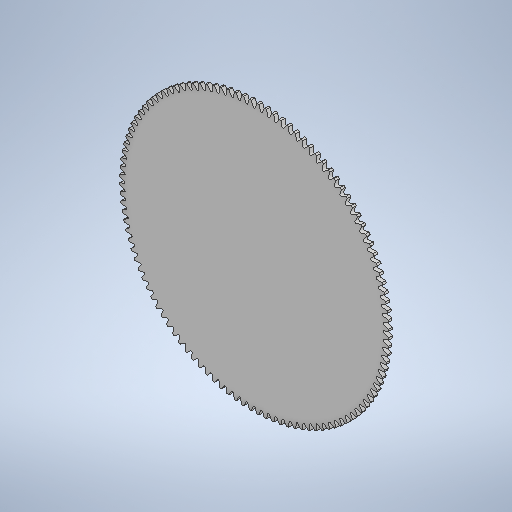
# Autodesk Inventor part: big gear 2.0
Saved by Autodesk Inventor 2025 (Build 290162010, 162A)
## iProperties
Created: 2025-09-06
Part Number: big gear 2.0
Material: Generic
Document SubType Name: Modeling
Designer: pokla
Density: 1 g/cm^3
Appearance: Default
Author: pokla
Autodesk Inventor part; units mm, degrees
ref_plane "YZ Plane" through (0, 0, 0) normal (1, 0, 0) x (0, 1, 0)
ref_plane "XZ Plane" through (0, 0, 0) normal (0, 1, 0) x (-1, 0, 0)
ref_plane "XY Plane" through (0, 0, 0) normal (0, 0, 1) x (1, 0, 0)
sketch "Sketch1" plane through (0, 0, 0) normal (0, 0, 1) x (1, 0, 0)
  spline S0 degree 3 poles (-14.9165, 712.3438) (-14.3601, 711.0686) (-13.2474, 708.5182) (-11.6564, 704.6592) (-10.1258, 700.7761) (-8.6597, 696.8679) (-7.2786, 692.9293) (-6.2598, 689.9687) (-5.6659, 687.9678) (-5.3327, 687.1621) (-4.9908, 686.5548) (-4.6754, 686.1384) (-4.3362, 685.7407) (-3.9402, 685.3992) (-3.5213, 685.0871) (-2.9134, 684.7464) (-2.2513, 684.5144) (-1.5656, 684.391) (-0.8692, 684.3646) (0, 684.3819) (0.8692, 684.3646) (1.5656, 684.391) (2.2513, 684.5144) (2.9134, 684.7464) (3.5213, 685.0871) (3.9402, 685.3992) (4.3362, 685.7407) (4.6754, 686.1384) (4.9908, 686.5548) (5.3327, 687.1621) (5.6659, 687.9678) (6.2598, 689.9687) (7.2786, 692.9293) (8.6597, 696.8679) (10.1258, 700.7761) (11.6564, 704.6592) (13.2474, 708.5182) (14.3601, 711.0686) (14.9165, 712.3438) knots 0 0 0 0 0.417378 0.834757 1.252136 1.669514 2.086891 2.50427 2.608615 2.712858 2.765031 2.8172 2.869347 2.921514 2.97367 3.025847 3.130039 3.182219 3.234379 3.338724 3.443069 3.495228 3.547409 3.6516 3.703778 3.755934 3.808101 3.860247 3.912416 3.964589 4.068833 4.173177 4.590556 5.007934 5.425312 5.842691 6.260069 6.677448 6.677448 6.677448 6.677448
  circle A0 centre (0, 0) radius 684.375 construction
  circle A1 centre (0, 0) radius 657.7848 construction
  circle A2 centre (0, 0) radius 700 construction
  circle A3 centre (0, 0) radius 712.5
  point P0 (-13.2604, 708.5127)
  point P1 (-11.6665, 704.6552)
  point P2 (-10.1366, 700.7719)
  point P3 (-8.6739, 696.8628)
  point P4 (-7.2824, 692.9279)
  point P5 (-5.9656, 688.9672)
  point P6 (-5.6486, 687.9731)
  point P7 (-5.2411, 687.0136)
  point P8 (-4.981, 686.5614)
  point P9 (-4.6714, 686.1415)
  point P10 (-4.3267, 685.7501)
  point P11 (-3.9363, 685.4041)
  point P12 (-3.5151, 685.0965)
  point P13 (-3.0605, 684.8405)
  point P14 (-2.0783, 684.4927)
  point P15 (-1.5643, 684.4032)
  point P16 (-1.0434, 684.3746)
  point P17 (0, 684.375)
  point P18 (1.0434, 684.3746)
  point P19 (1.5643, 684.4032)
  point P20 (2.0783, 684.4927)
  point P21 (3.0605, 684.8405)
  point P22 (3.5151, 685.0965)
  point P23 (3.9363, 685.4041)
  point P24 (4.3267, 685.7501)
  point P25 (4.6714, 686.1415)
  point P26 (4.981, 686.5614)
  point P27 (5.2411, 687.0136)
  point P28 (5.6486, 687.9731)
  point P29 (5.9656, 688.9672)
  point P30 (7.2824, 692.9279)
  point P31 (8.6739, 696.8628)
  point P32 (10.1366, 700.7719)
  point P33 (11.6665, 704.6552)
  point P34 (13.2604, 708.5127)
  constraints: 4 centre point, 2 point on circle, 79 other
extrude "Extrusion1" add sketch "Sketch1" against normal blind 20
extrude "Extrusion2" cut sketch "Sketch1" against normal through all contours A3 S0 picked at (-0.9229, 701.9967)
pattern_circular "Circular Pattern1" count 112 over 360 about axis through (0, 0, -10) along (0, 0, 1) of "Extrusion2"
sketch "Sketch2" plane through (0, 0, 0) normal (0, 0, 1) x (1, 0, 0)
  circle A0 centre (0, 0) radius 360
  line L0 (0, 0) -> (0, 360) construction
  line L1 (0, 0) -> (76.6258, 680.0718)
  line L2 (0, 0) -> (-76.6258, 680.0718)
  arc A1 (25.0484, 712.0596) -> (14.9165, 712.3438) centre (0, 0) ccw projected
  arc A2 (-14.9165, 712.3438) -> (-25.0484, 712.0596) centre (0, 0) ccw projected
  arc A3 (-54.8344, 710.3868) -> (-64.9345, 709.5349) centre (0, 0) ccw projected
  arc A4 (-94.5799, 706.1947) -> (-104.6163, 704.7778) centre (0, 0) ccw projected
  arc A5 (-134.0277, 699.7805) -> (-143.9689, 697.8031) centre (0, 0) ccw projected
  arc A6 (-173.0539, 691.1647) -> (-182.8686, 688.6329) centre (0, 0) ccw projected
  arc A7 (-211.5356, 680.3741) -> (-221.1928, 677.2961) centre (0, 0) ccw projected
  arc A8 (-249.3517, 667.4429) -> (-258.8212, 663.8282) centre (0, 0) ccw projected
  arc A9 (-286.3832, 652.4116) -> (-295.6351, 648.2716) centre (0, 0) ccw projected
  arc A10 (-322.5137, 635.3276) -> (-331.5189, 630.6754) centre (0, 0) ccw projected
  arc A11 (-357.6294, 616.2446) -> (-366.3596, 611.0948) centre (0, 0) ccw projected
  arc A12 (-391.6199, 595.2227) -> (-400.0476, 589.5915) centre (0, 0) ccw projected
  arc A13 (-424.3782, 572.328) -> (-432.4769, 566.2331) centre (0, 0) ccw projected
  arc A14 (-455.8013, 547.6326) -> (-463.5455, 541.0931) centre (0, 0) ccw projected
  arc A15 (-485.7902, 521.2141) -> (-493.1556, 514.2507) centre (0, 0) ccw projected
  arc A16 (-514.2507, 493.1556) -> (-521.2141, 485.7902) centre (0, 0) ccw projected
  arc A17 (-541.0931, 463.5455) -> (-547.6326, 455.8013) centre (0, 0) ccw projected
  arc A18 (-566.2331, 432.4769) -> (-572.328, 424.3782) centre (0, 0) ccw projected
  arc A19 (-589.5915, 400.0476) -> (-595.2227, 391.6199) centre (0, 0) ccw projected
  arc A20 (-611.0948, 366.3596) -> (-616.2446, 357.6294) centre (0, 0) ccw projected
  arc A21 (-630.6754, 331.5189) -> (-635.3276, 322.5137) centre (0, 0) ccw projected
  arc A22 (-648.2716, 295.6351) -> (-652.4116, 286.3832) centre (0, 0) ccw projected
  arc A23 (-663.8282, 258.8212) -> (-667.4429, 249.3517) centre (0, 0) ccw projected
  arc A24 (-677.2961, 221.1928) -> (-680.3741, 211.5356) centre (0, 0) ccw projected
  arc A25 (-688.6329, 182.8686) -> (-691.1647, 173.0539) centre (0, 0) ccw projected
  arc A26 (-697.8031, 143.9689) -> (-699.7805, 134.0277) centre (0, 0) ccw projected
  arc A27 (-704.7778, 104.6163) -> (-706.1947, 94.5799) centre (0, 0) ccw projected
  arc A28 (-709.5349, 64.9345) -> (-710.3868, 54.8344) centre (0, 0) ccw projected
  arc A29 (-712.0596, 25.0484) -> (-712.3438, 14.9165) centre (0, 0) ccw projected
  arc A30 (-712.3438, -14.9165) -> (-712.0596, -25.0484) centre (0, 0) ccw projected
  arc A31 (-710.3868, -54.8344) -> (-709.5349, -64.9345) centre (0, 0) ccw projected
  arc A32 (-706.1947, -94.5799) -> (-704.7778, -104.6163) centre (0, 0) ccw projected
  arc A33 (-699.7805, -134.0277) -> (-697.8031, -143.9689) centre (0, 0) ccw projected
  arc A34 (-691.1647, -173.0539) -> (-688.6329, -182.8686) centre (0, 0) ccw projected
  arc A35 (-680.3741, -211.5356) -> (-677.2961, -221.1928) centre (0, 0) ccw projected
  arc A36 (-667.4429, -249.3517) -> (-663.8282, -258.8212) centre (0, 0) ccw projected
  arc A37 (-652.4116, -286.3832) -> (-648.2716, -295.6351) centre (0, 0) ccw projected
  arc A38 (-635.3276, -322.5137) -> (-630.6754, -331.5189) centre (0, 0) ccw projected
  arc A39 (-616.2446, -357.6294) -> (-611.0948, -366.3596) centre (0, 0) ccw projected
  arc A40 (-595.2227, -391.6199) -> (-589.5915, -400.0476) centre (0, 0) ccw projected
  arc A41 (-572.328, -424.3782) -> (-566.2331, -432.4769) centre (0, 0) ccw projected
  arc A42 (-547.6326, -455.8013) -> (-541.0931, -463.5455) centre (0, 0) ccw projected
  arc A43 (-521.2141, -485.7902) -> (-514.2507, -493.1556) centre (0, 0) ccw projected
  arc A44 (-493.1556, -514.2507) -> (-485.7902, -521.2141) centre (0, 0) ccw projected
  arc A45 (-463.5455, -541.0931) -> (-455.8013, -547.6326) centre (0, 0) ccw projected
  arc A46 (-432.4769, -566.2331) -> (-424.3782, -572.328) centre (0, 0) ccw projected
  arc A47 (-400.0476, -589.5915) -> (-391.6199, -595.2227) centre (0, 0) ccw projected
  arc A48 (-366.3596, -611.0948) -> (-357.6294, -616.2446) centre (0, 0) ccw projected
  arc A49 (-331.5189, -630.6754) -> (-322.5137, -635.3276) centre (0, 0) ccw projected
  arc A50 (-295.6351, -648.2716) -> (-286.3832, -652.4116) centre (0, 0) ccw projected
  arc A51 (-258.8212, -663.8282) -> (-249.3517, -667.4429) centre (0, 0) ccw projected
  arc A52 (-221.1928, -677.2961) -> (-211.5356, -680.3741) centre (0, 0) ccw projected
  arc A53 (-182.8686, -688.6329) -> (-173.0539, -691.1647) centre (0, 0) ccw projected
  arc A54 (-143.9689, -697.8031) -> (-134.0277, -699.7805) centre (0, 0) ccw projected
  arc A55 (-104.6163, -704.7778) -> (-94.5799, -706.1947) centre (0, 0) ccw projected
  arc A56 (-64.9345, -709.5349) -> (-54.8344, -710.3868) centre (0, 0) ccw projected
  arc A57 (-25.0484, -712.0596) -> (-14.9165, -712.3438) centre (0, 0) ccw projected
  arc A58 (14.9165, -712.3438) -> (25.0484, -712.0596) centre (0, 0) ccw projected
  arc A59 (54.8344, -710.3868) -> (64.9345, -709.5349) centre (0, 0) ccw projected
  arc A60 (94.5799, -706.1947) -> (104.6163, -704.7778) centre (0, 0) ccw projected
  arc A61 (134.0277, -699.7805) -> (143.9689, -697.8031) centre (0, 0) ccw projected
  arc A62 (173.0539, -691.1647) -> (182.8686, -688.6329) centre (0, 0) ccw projected
  arc A63 (211.5356, -680.3741) -> (221.1928, -677.2961) centre (0, 0) ccw projected
  arc A64 (249.3517, -667.4429) -> (258.8212, -663.8282) centre (0, 0) ccw projected
  arc A65 (286.3832, -652.4116) -> (295.6351, -648.2716) centre (0, 0) ccw projected
  arc A66 (322.5137, -635.3276) -> (331.5189, -630.6754) centre (0, 0) ccw projected
  arc A67 (357.6294, -616.2446) -> (366.3596, -611.0948) centre (0, 0) ccw projected
  arc A68 (391.6199, -595.2227) -> (400.0476, -589.5915) centre (0, 0) ccw projected
  arc A69 (424.3782, -572.328) -> (432.4769, -566.2331) centre (0, 0) ccw projected
  arc A70 (455.8013, -547.6326) -> (463.5455, -541.0931) centre (0, 0) ccw projected
  arc A71 (485.7902, -521.2141) -> (493.1556, -514.2507) centre (0, 0) ccw projected
  arc A72 (514.2507, -493.1556) -> (521.2141, -485.7902) centre (0, 0) ccw projected
  arc A73 (541.0931, -463.5455) -> (547.6326, -455.8013) centre (0, 0) ccw projected
  arc A74 (566.2331, -432.4769) -> (572.328, -424.3782) centre (0, 0) ccw projected
  arc A75 (589.5915, -400.0476) -> (595.2227, -391.6199) centre (0, 0) ccw projected
  arc A76 (611.0948, -366.3596) -> (616.2446, -357.6294) centre (0, 0) ccw projected
  arc A77 (630.6754, -331.5189) -> (635.3276, -322.5137) centre (0, 0) ccw projected
  arc A78 (648.2716, -295.6351) -> (652.4116, -286.3832) centre (0, 0) ccw projected
  arc A79 (663.8282, -258.8212) -> (667.4429, -249.3517) centre (0, 0) ccw projected
  arc A80 (677.2961, -221.1928) -> (680.3741, -211.5356) centre (0, 0) ccw projected
  arc A81 (688.6329, -182.8686) -> (691.1647, -173.0539) centre (0, 0) ccw projected
  arc A82 (697.8031, -143.9689) -> (699.7805, -134.0277) centre (0, 0) ccw projected
  arc A83 (704.7778, -104.6163) -> (706.1947, -94.5799) centre (0, 0) ccw projected
  arc A84 (709.5349, -64.9345) -> (710.3868, -54.8344) centre (0, 0) ccw projected
  arc A85 (712.0596, -25.0484) -> (712.3438, -14.9165) centre (0, 0) ccw projected
  arc A86 (712.3438, 14.9165) -> (712.0596, 25.0484) centre (0, 0) ccw projected
  arc A87 (710.3868, 54.8344) -> (709.5349, 64.9345) centre (0, 0) ccw projected
  arc A88 (706.1947, 94.5799) -> (704.7778, 104.6163) centre (0, 0) ccw projected
  arc A89 (699.7805, 134.0277) -> (697.8031, 143.9689) centre (0, 0) ccw projected
  arc A90 (691.1647, 173.0539) -> (688.6329, 182.8686) centre (0, 0) ccw projected
  arc A91 (680.3741, 211.5356) -> (677.2961, 221.1928) centre (0, 0) ccw projected
  arc A92 (667.4429, 249.3517) -> (663.8282, 258.8212) centre (0, 0) ccw projected
  arc A93 (652.4116, 286.3832) -> (648.2716, 295.6351) centre (0, 0) ccw projected
  arc A94 (635.3276, 322.5137) -> (630.6754, 331.5189) centre (0, 0) ccw projected
  arc A95 (616.2446, 357.6294) -> (611.0948, 366.3596) centre (0, 0) ccw projected
  arc A96 (595.2227, 391.6199) -> (589.5915, 400.0476) centre (0, 0) ccw projected
  arc A97 (572.328, 424.3782) -> (566.2331, 432.4769) centre (0, 0) ccw projected
  arc A98 (547.6326, 455.8013) -> (541.0931, 463.5455) centre (0, 0) ccw projected
  arc A99 (521.2141, 485.7902) -> (514.2507, 493.1556) centre (0, 0) ccw projected
  arc A100 (493.1556, 514.2507) -> (485.7902, 521.2141) centre (0, 0) ccw projected
  arc A101 (463.5455, 541.0931) -> (455.8013, 547.6326) centre (0, 0) ccw projected
  arc A102 (432.4769, 566.2331) -> (424.3782, 572.328) centre (0, 0) ccw projected
  arc A103 (400.0476, 589.5915) -> (391.6199, 595.2227) centre (0, 0) ccw projected
  arc A104 (366.3596, 611.0948) -> (357.6294, 616.2446) centre (0, 0) ccw projected
  arc A105 (331.5189, 630.6754) -> (322.5137, 635.3276) centre (0, 0) ccw projected
  arc A106 (295.6351, 648.2716) -> (286.3832, 652.4116) centre (0, 0) ccw projected
  arc A107 (258.8212, 663.8282) -> (249.3517, 667.4429) centre (0, 0) ccw projected
  arc A108 (221.1928, 677.2961) -> (211.5356, 680.3741) centre (0, 0) ccw projected
  arc A109 (182.8686, 688.6329) -> (173.0539, 691.1647) centre (0, 0) ccw projected
  arc A110 (143.9689, 697.8031) -> (134.0277, 699.7805) centre (0, 0) ccw projected
  arc A111 (104.6163, 704.7778) -> (94.5799, 706.1947) centre (0, 0) ccw projected
  arc A112 (64.9345, 709.5349) -> (54.8344, 710.3868) centre (0, 0) ccw projected
  point P0 (40.3073, 357.7364)
  point P1 (-40.3073, 357.7364)
  dimension "d7" = 720
  dimension "d8" = 12.857
  constraints: 6 end point, 2 horizontal alignment, 2 vertical alignment, 1 coincident, 1 vertical, 114 other
  measures "d8" angle of L1 L2
extrude "Extrusion3" [suppressed]
equation "\"d0\" = FaceWidth"
equation "\"d7\" = Шстр_диам_внутр"
equation "\"Module\" = 12.5"
equation "\"PressureAngle\" = 20deg"
equation "\"UnitProfileClearance\" = 0.25"
equation "\"UnitRoundRadius\" = 0.35"
equation "\"HeadDiameter\" = 1425"
equation "\"RootDiameter\" = 1368.75"
equation "\"BaseDiameter\" = 1315.56967"
equation "\"FaceWidth\" = 20"
equation "\"HelixAngle\" = 0"
equation "\"UnitCorrection\" = 0"
equation "\"UnitAddendumModification\" = 0"
equation "\"CircularPitch\" = 39.269908"
equation "\"UnitBacklashShift\" = 0"
equation "\"TotalToolShift\" = 0"
equation "\"IsInternal\" = 0"
equation "\"Шстр_диам_внутр\" = 720"
body "Solid1"
